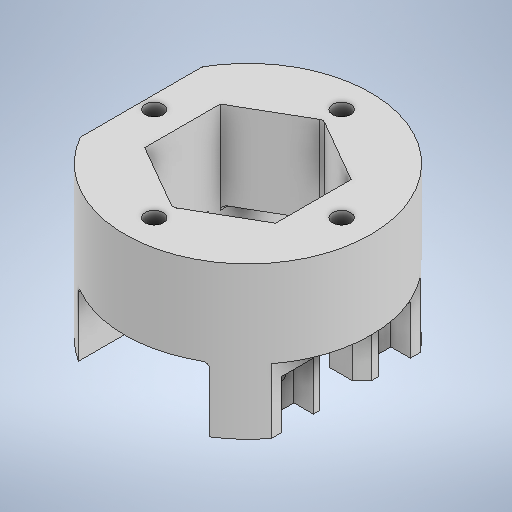
# Autodesk Inventor part: Platform Frame Mount Adapter
Saved by Autodesk Inventor 2025 (Build 290162000, 162)
## iProperties
Created: 2025-05-21
Part Number: Platform Frame Mount Adapter
Material: Generic
Document SubType Name: Modeling
Designer: mumin
Density: 1 g/cm^3
Appearance: Default
Author: mumin
Autodesk Inventor part; units mm, degrees
ref_plane "YZ Plane" through (0, 0, 0) normal (1, 0, 0) x (0, 1, 0)
ref_plane "XZ Plane" through (0, 0, 0) normal (0, 1, 0) x (-1, 0, 0)
ref_plane "XY Plane" through (0, 0, 0) normal (0, 0, 1) x (1, 0, 0)
sketch "Sketch1" plane through (0, 0, 0) normal (0, 1, 0) x (-1, 0, 0)
  arc A0 (36, 19.6214) -> (36, -19.6214) centre (0, 0) ccw
  line L0 (36, 19.6214) -> (36, -19.6214)
  line L1 (33, -18.8414) -> (33, 18.8414)
  arc A1 (33, 18.8414) -> (33, -18.8414) centre (0, 0) ccw
  dimension "d0" = 82
  dimension "d1" = 36
  dimension "d2" = 3
  constraints: 4 end point, 4 point on circle, 2 centre point, 1 coincident, 1 vertical, 1 other
  measures "d0" diameter of A0
  measures "d1" distance from line of point (0, 0) L0
  measures "d2" distance between parallel lines of L0 L1
extrude "Key Shape" add sketch "Sketch1" against normal blind 27 contours A1 L1
sketch "Sketch2" plane through (0, -27, 0) normal (0, -1, 0) x (1, 0, 0)
  line L0 (20.25, -32.1549) -> (20.25, 32.1549)
  arc A0 (-33, -18.8414) -> (-33, 18.8414) centre (0, 0) ccw projected
  line L1 (30.25, 22.9986) -> (30.25, -22.9986)
  line L2 (30.25, 5) -> (20.25, 5)
  line L3 (20.25, 5) -> (20.25, -5)
  line L4 (20.25, -5) -> (30.25, -5)
  line L5 (30.25, -5) -> (30.25, 5)
  point P0 (20.25, 0)
  point P1 (20.25, 5)
  point P2 (30.25, -5)
  dimension "d5" = 20.25
  dimension "d6" = 10
  dimension "d40" = 10
  constraints: 12 end point, 4 point on circle, 2 midpoint, 2 parallel, 2 point on line, 1 horizontal, 1 perpendicular, 1 vertical
  measures "d5" distance from line of point (0, 0) L0
  measures "d6" distance between parallel lines of L0 L1
  measures "d40" distance between parallel lines of L2 L4
extrude "Side Walls" add sketch "Sketch2" along normal blind 20 contours L0 L4 L1 A0 | L0 A0 L1 L2
sketch "Sketch3" plane through (0, 0, 0) normal (0, 1, 0) x (1, 0, 0)
  line L0 (-47.2, 0) -> (52.2, 0) projected
  point P0 (0, 0)
  point P1 (-29, 0)
  dimension "d16" = 29
  constraints: 1 point on line
  measures "d16" distance of point (-29, 0) point (0, 0)
hole "M5 Holes" at (-29, 0, 0) direction (0, -1, 0) diameter 5.6 depth 27 tip angle 118
pattern_circular "Circular Pattern1" count 4 over 360 about axis through (0, -10, 0) along (0, 1, 0) of "M5 Holes"
sketch "Sketch4" plane through (30.25, -27, 22.9986) normal (1, 0, 0) x (0, 0, -1)
  line L0 (45.9973, -20) -> (0, -20) projected
  line L1 (2.9986, -20) -> (12.9986, -20)
  line L2 (12.9986, -20) -> (12.9986, -5)
  line L3 (12.9986, -5) -> (2.9986, -5)
  line L4 (2.9986, -5) -> (2.9986, -20)
  line L5 (22.9986, -29.4) -> (22.9986, 36.4) projected
  point P0 (22.9986, 27)
  point P1 (7.9986, -5)
  point P2 (12.9986, -20)
  point P3 (12.9986, -20)
  dimension "d20" = 10
  dimension "d21" = 15
  dimension "d22" = 15
  constraints: 8 end point, 2 parallel, 1 horizontal, 1 midpoint, 1 perpendicular, 1 point on line
  measures "d20" distance of L2.end L3.end
  measures "d21" distance of L1.end L2.end
  measures "d22" distance from line of L5 point (7.999, -5)
extrude "M4 Bolt Seats" cut sketch "Sketch4" against normal blind 6
sketch "Sketch5" plane through (24.25, -27, 22.9986) normal (1, 0, 0) x (0, 0, -1)
  line L0 (22.9986, -29.4) -> (22.9986, 36.4) projected
  line L1 (45.9973, -20) -> (12.9986, -20) projected
  point P0 (22.9986, 27)
  point P1 (7.9986, -10)
  dimension "d32" = 15
  dimension "d33" = 10
  measures "d32" distance from line of L0 point (7.999, -10)
  measures "d33" distance from line of L1 point (7.999, -10)
hole "M4 Holes" at (24.25, -37, 15) direction (-1, 0, 0) diameter 5.5 depth 4 tip angle 118
mirror "Mirror1" about plane through (0, 0, 0) normal (0, 0, 1) of "M4 Bolt Seats", "M4 Holes"
mirror "Mirror2" about plane through (0, 0, 0) normal (1, 0, 0) of "Side Walls", "M4 Bolt Seats", "M4 Holes", "Mirror1"
chamfer "Chamfer1" distance 3 angle 45 4 edges at (30.25, -37, 5) (30.25, -37, -5) (-20.25, -37, 5) (-20.25, -37, -5)
sketch "Sketch6" plane through (0, -27, 0) normal (0, -1, 0) x (1, 0, 0)
  circle A0 centre (29, 0) radius 2.8 projected
  line L0 (33.7631, 0) -> (31.3816, -4.125)
  line L1 (31.3816, -4.125) -> (26.6184, -4.125)
  line L2 (26.6184, -4.125) -> (24.2369, 0)
  line L3 (24.2369, 0) -> (26.6184, 4.125)
  line L4 (26.6184, 4.125) -> (31.3816, 4.125)
  line L5 (31.3816, 4.125) -> (33.7631, 0)
  point P0 (0, 0)
  dimension "d46" = 8.25
  constraints: 12 end point, 1 coincident, 13 other
  measures "d46" distance between parallel lines of L1 L4
extrude "Nut Seats" cut sketch "Sketch6" against normal blind 4
pattern_circular "Circular Pattern2" count 4 over 360 about axis through (0, -10, 0) along (0, 1, 0) of "Nut Seats"
sketch "Sketch7" plane through (0, -27, 0) normal (0, -1, 0) x (1, 0, 0)
  line L0 (0, 23.3827) -> (20.25, 11.6913)
  line L1 (20.25, 11.6913) -> (20.25, -11.6913)
  line L2 (20.25, -11.6913) -> (0, -23.3827)
  line L3 (0, -23.3827) -> (-20.25, -11.6913)
  line L4 (-20.25, -11.6913) -> (-20.25, 11.6913)
  line L5 (-20.25, 11.6913) -> (0, 23.3827)
  point P0 (0, 0)
  point P1 (0, 0)
  dimension "d52" = 40.5
  constraints: 12 end point, 1 coincident, 13 other
  measures "d52" distance between parallel lines of L4 L1
extrude "Hollow Center" cut sketch "Sketch7" against normal up to surface (27 mm away)
fillet "Fillet9" radius 1.5 6 edges at (-20.25, -27, 21.9231) (-20.25, -27, -21.9231) (20.25, -27, 21.9231) (20.25, -27, -21.9231) (0, -13.5, -23.3827) (0, -13.5, 23.3827)
body "Solid1"
